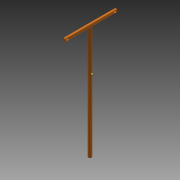
# Autodesk Inventor part: 1
Saved by Autodesk Inventor 2015 (Build 190159000, 159)
## iProperties
Created: 2016-03-10
Part Number: 1
Material: Złote
Document SubType Name: Modeling
Designer: Arek
Density: 19.3 g/cm^3
Appearance: Gorący metal 1600F
Mass: 21314.3 g
Surface Area: 1530.25 cm^2
Volume: 1104.37 cm^3
Author: Arek
Autodesk Inventor part; units mm, degrees
ref_plane "XZ Plane" through (0, 0, 0) normal (0, 1, 0) x (-1, 0, 0)
ref_plane "XY Plane" through (0, 0, 0) normal (0, 0, 1) x (1, 0, 0)
sketch "Szkic1" plane through (0, 0, 0) normal (0, 1, 0) x (-1, 0, 0)
  circle A0 centre (0, 0) radius 15
  dimension "d0" = 30
  constraints: 1 centre point, 1 coincident
  measures "d0" diameter of A0
extrude "Wyciągnięcie proste1" add sketch "Szkic1" along normal blind 400
sketch "Szkic2" plane through (0, 0, 0) normal (0, 0, 1) x (1, 0, 0)
  point P0 (0, 0)
sketch "Szkic3" plane through (0, 0, 0) normal (0, 0, 1) x (1, 0, 0)
  circle A0 centre (0, 400) radius 15
  point P0 (0, 0)
  dimension "d3" = 30
  constraints: 1 centre point
  measures "d3" diameter of A0
extrude "Wyciągnięcie proste2" add sketch "Szkic3" along normal mid plane 500
fillet "Zaokrąglenie1" radius 4 4 edges at (-10.6066, 389.3934, -10.6066) (10.6066, 389.3934, -10.6066) (10.6066, 389.3934, 10.6066) (-10.6066, 389.3934, 10.6066)
ref_plane "Płaszczyzna konstrukcyjna1" through (15, 0, 0) normal (1, 0, 0) x (0, 1, 0)
sketch "Szkic4" plane through (15, 0, 0) normal (1, 0, 0) x (0, 1, 0)
  line L0 (400, 0) -> (400, 0) projected
  line L1 (400, 0) -> (400, 0) projected
  line L2 (415, 250) -> (385, 250) projected
  line L3 (385, -250) -> (415, -250) projected
  line L4 (400, 0) -> (400, 0) projected
  line L5 (400, 0) -> (400, 0) projected
  line L6 (0, 15) -> (0, -15) projected
  line L7 (0, 15) -> (381, 15) projected
  line L8 (0, -15) -> (381, -15) projected
  line L9 (385, -250) -> (385, 250) projected
  line L10 (415, -250) -> (415, 250) projected
  circle A0 centre (400, 230) radius 10
  point P0 (0, 0)
  dimension "d8" = 20
  dimension "d9" = 20
  constraints: 1 centre point
  measures "d8" diameter of A0
  measures "d9" distance from line of A0.centre L2
extrude "Wyciągnięcie proste3" cut sketch "Szkic4" against normal through all contours A0
mirror "Odbicie lustrzane1" about plane through (0, 0, 0) normal (0, 0, 1) of "Wyciągnięcie proste3"
sketch "Szkic5" plane through (0, 0, 0) normal (0, -1, 0) x (1, 0, 0)
  circle A0 centre (0, 0) radius 15 projected
extrude "Wyciągnięcie proste4" add sketch "Szkic5" along normal blind 700
sketch "Szkic6" plane through (15, 0, 0) normal (1, 0, 0) x (0, 1, 0)
  point P0 (0, 0)
